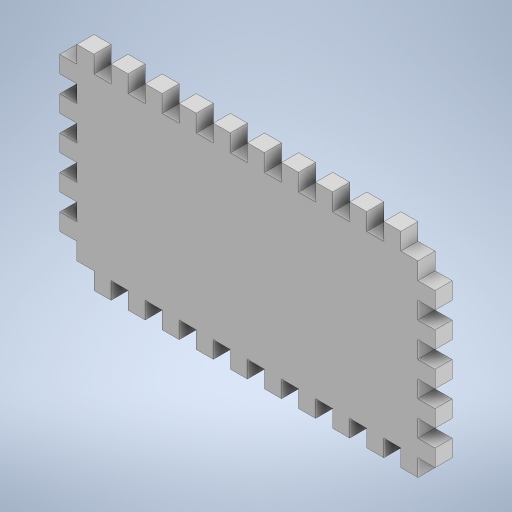
# Autodesk Inventor part: backside
Saved by Autodesk Inventor 2024 (Build 280153000, 153)
## iProperties
Created: 2024-04-15
Part Number: backside
Material: Generic
Document SubType Name: Modeling
Designer: srika
Density: 1 g/cm^3
Appearance: Default
Author: srika
Autodesk Inventor part; units mm, degrees
ref_plane "YZ Plane" through (0, 0, 0) normal (1, 0, 0) x (0, 1, 0)
ref_plane "XZ Plane" through (0, 0, 0) normal (0, 1, 0) x (-1, 0, 0)
ref_plane "XY Plane" through (0, 0, 0) normal (0, 0, 1) x (1, 0, 0)
sketch "Sketch2" plane through (0, 0, 0) normal (0, 0, 1) x (1, 0, 0)
  line L0 (0, 0) -> (5, 0)
  line L1 (5, 0) -> (5, 5)
  line L2 (5, 5) -> (0, 5)
  line L3 (0, 5) -> (0, 0)
  line L4 (5, 5) -> (105, 5)
  line L5 (105, 5) -> (105, 55)
  line L6 (105, 55) -> (5, 55)
  line L7 (5, 55) -> (5, 5)
  line L8 (105, 55) -> (110, 55)
  line L9 (110, 55) -> (110, 60)
  line L10 (110, 60) -> (105, 60)
  line L11 (105, 60) -> (105, 55)
  line L12 (100, 60) -> (95, 60)
  line L13 (100, 55) -> (100, 60)
  line L14 (95, 60) -> (95, 55)
  line L15 (90, 60) -> (85, 60)
  line L16 (90, 55) -> (90, 60)
  line L17 (85, 60) -> (85, 55)
  line L18 (80, 60) -> (75, 60)
  line L19 (80, 55) -> (80, 60)
  line L20 (75, 60) -> (75, 55)
  line L21 (70, 60) -> (65, 60)
  line L22 (70, 55) -> (70, 60)
  line L23 (65, 60) -> (65, 55)
  line L24 (60, 60) -> (55, 60)
  line L25 (60, 55) -> (60, 60)
  line L26 (55, 60) -> (55, 55)
  line L27 (50, 60) -> (45, 60)
  line L28 (50, 55) -> (50, 60)
  line L29 (45, 60) -> (45, 55)
  line L30 (40, 60) -> (35, 60)
  line L31 (40, 55) -> (40, 60)
  line L32 (35, 60) -> (35, 55)
  line L33 (30, 60) -> (25, 60)
  line L34 (30, 55) -> (30, 60)
  line L35 (25, 60) -> (25, 55)
  line L36 (20, 60) -> (15, 60)
  line L37 (20, 55) -> (20, 60)
  line L38 (15, 60) -> (15, 55)
  line L39 (10, 60) -> (5, 60)
  line L40 (10, 55) -> (10, 60)
  line L41 (5, 60) -> (5, 55)
  line L42 (105, 50) -> (105, 45)
  line L43 (110, 45) -> (110, 50)
  line L44 (110, 50) -> (105, 50)
  line L45 (105, 45) -> (110, 45)
  line L46 (105, 40) -> (105, 35)
  line L47 (110, 35) -> (110, 40)
  line L48 (110, 40) -> (105, 40)
  line L49 (105, 35) -> (110, 35)
  line L50 (105, 30) -> (105, 25)
  line L51 (110, 25) -> (110, 30)
  line L52 (110, 30) -> (105, 30)
  line L53 (105, 25) -> (110, 25)
  line L54 (105, 20) -> (105, 15)
  line L55 (110, 15) -> (110, 20)
  line L56 (110, 20) -> (105, 20)
  line L57 (105, 15) -> (110, 15)
  line L58 (105, 10) -> (105, 5)
  line L59 (110, 5) -> (110, 10)
  line L60 (110, 10) -> (105, 10)
  line L61 (105, 5) -> (110, 5)
  line L62 (0, 10) -> (5, 10)
  line L63 (5, 10) -> (5, 15)
  line L64 (5, 15) -> (0, 15)
  line L65 (0, 15) -> (0, 10)
  line L66 (0, 20) -> (5, 20)
  line L67 (5, 20) -> (5, 25)
  line L68 (5, 25) -> (0, 25)
  line L69 (0, 25) -> (0, 20)
  line L70 (0, 30) -> (5, 30)
  line L71 (5, 30) -> (5, 35)
  line L72 (5, 35) -> (0, 35)
  line L73 (0, 35) -> (0, 30)
  line L74 (0, 40) -> (5, 40)
  line L75 (5, 40) -> (5, 45)
  line L76 (5, 45) -> (0, 45)
  line L77 (0, 45) -> (0, 40)
  line L78 (0, 50) -> (5, 50)
  line L79 (5, 50) -> (5, 55)
  line L80 (5, 55) -> (0, 55)
  line L81 (0, 55) -> (0, 50)
  line L82 (15, 5) -> (10, 5)
  line L83 (10, 0) -> (15, 0)
  line L84 (15, 0) -> (15, 5)
  line L85 (10, 5) -> (10, 0)
  line L86 (25, 5) -> (20, 5)
  line L87 (20, 0) -> (25, 0)
  line L88 (25, 0) -> (25, 5)
  line L89 (20, 5) -> (20, 0)
  line L90 (35, 5) -> (30, 5)
  line L91 (30, 0) -> (35, 0)
  line L92 (35, 0) -> (35, 5)
  line L93 (30, 5) -> (30, 0)
  line L94 (45, 5) -> (40, 5)
  line L95 (40, 0) -> (45, 0)
  line L96 (45, 0) -> (45, 5)
  line L97 (40, 5) -> (40, 0)
  line L98 (55, 5) -> (50, 5)
  line L99 (50, 0) -> (55, 0)
  line L100 (55, 0) -> (55, 5)
  line L101 (50, 5) -> (50, 0)
  line L102 (65, 5) -> (60, 5)
  line L103 (60, 0) -> (65, 0)
  line L104 (65, 0) -> (65, 5)
  line L105 (60, 5) -> (60, 0)
  line L106 (75, 5) -> (70, 5)
  line L107 (70, 0) -> (75, 0)
  line L108 (75, 0) -> (75, 5)
  line L109 (70, 5) -> (70, 0)
  line L110 (85, 5) -> (80, 5)
  line L111 (80, 0) -> (85, 0)
  line L112 (85, 0) -> (85, 5)
  line L113 (80, 5) -> (80, 0)
  line L114 (95, 5) -> (90, 5)
  line L115 (90, 0) -> (95, 0)
  line L116 (95, 0) -> (95, 5)
  line L117 (90, 5) -> (90, 0)
  line L118 (105, 5) -> (100, 5)
  line L119 (100, 0) -> (105, 0)
  line L120 (105, 0) -> (105, 5)
  line L121 (100, 5) -> (100, 0)
  circle A0 centre (12.3298, 40) radius 3.5
  line L122 (6.3298, 15) -> (18.3298, 15)
  line L123 (18.3298, 15) -> (18.3298, 45)
  line L124 (18.3298, 45) -> (6.3298, 45)
  line L125 (6.3298, 45) -> (6.3298, 15)
  line L126 (6.3298, 15) -> (18.3298, 45) construction
  line L127 (18.3298, 15) -> (6.3298, 45) construction
  line L128 (19, 15) -> (31, 15)
  circle A1 centre (25, 40) radius 3.5
  line L129 (19, 45) -> (19, 15)
  line L130 (31, 15) -> (31, 45)
  line L131 (19, 15) -> (31, 45) construction
  line L132 (31, 15) -> (19, 45) construction
  line L133 (31, 45) -> (19, 45)
  line L134 (31.5, 15) -> (43.5, 15)
  circle A2 centre (37.5, 40) radius 3.5
  line L135 (31.5, 45) -> (31.5, 15)
  line L136 (43.5, 15) -> (43.5, 45)
  line L137 (31.5, 15) -> (43.5, 45) construction
  line L138 (43.5, 15) -> (31.5, 45) construction
  line L139 (43.5, 45) -> (31.5, 45)
  line L140 (44.1702, 45) -> (44.1702, 15)
  line L141 (56.1702, 15) -> (56.1702, 45)
  line L142 (56.1702, 15) -> (44.1702, 45) construction
  line L143 (44.1702, 15) -> (56.1702, 45) construction
  line L144 (56.1702, 45) -> (44.1702, 45)
  circle A3 centre (50.1702, 40) radius 3.5
  line L145 (44.1702, 15) -> (56.1702, 15)
  line L146 (57.3642, 14.8119) -> (69.3642, 14.8119)
  line L147 (57.3642, 44.8119) -> (57.3642, 14.8119)
  line L148 (69.3642, 44.8119) -> (57.3642, 44.8119)
  line L149 (57.3642, 14.8119) -> (69.3642, 44.8119) construction
  line L150 (69.3642, 14.8119) -> (57.3642, 44.8119) construction
  line L151 (69.3642, 14.8119) -> (69.3642, 44.8119)
  circle A4 centre (63.3642, 39.8119) radius 3.5
  line L152 (75, 15) -> (100, 15)
  line L153 (100, 15) -> (100, 45)
  line L154 (100, 45) -> (75, 45)
  line L155 (75, 45) -> (75, 15)
  line L156 (75, 15) -> (100, 45) construction
  line L157 (100, 15) -> (75, 45) construction
  line L158 (82.75, 38.25) -> (92.25, 38.25)
  line L159 (92.25, 38.25) -> (92.25, 41.75)
  line L160 (92.25, 41.75) -> (82.75, 41.75)
  line L161 (82.75, 41.75) -> (82.75, 38.25)
  line L162 (82.75, 38.25) -> (92.25, 41.75) construction
  line L163 (92.25, 38.25) -> (82.75, 41.75) construction
  point P0 (87.5, 30)
  point P1 (87.5, 40)
  dimension "d0" = 5
  dimension "d1" = 5
  dimension "d4" = 5
  dimension "d5" = 5
  dimension "d8" = 10
  dimension "d15" = 10
  dimension "d22" = 10
  dimension "d29" = 10
  dimension "d37" = 7
  dimension "d38" = 12
  dimension "d39" = 30
  dimension "d51" = 7
  dimension "d52" = 12
  dimension "d53" = 30
  dimension "d54" = 7
  dimension "d55" = 12
  dimension "d56" = 30
  dimension "d57" = 7
  dimension "d58" = 12
  dimension "d59" = 30
  dimension "d60" = 7
  dimension "d61" = 12
  dimension "d62" = 30
  dimension "d63" = 25
  dimension "d64" = 30
  dimension "d65" = 9.5
  dimension "d66" = 3.5
  constraints: 324 end point, 80 horizontal alignment, 59 parallel, 30 collinear, 9 horizontal, 9 perpendicular, 5 centre point, 4 midpoint, 3 vertical, 86 other
  measures "d0" distance of L2.end L1.end
  measures "d1" distance of L1.end L0.end
  measures "d4" distance of L10.end L9.end
  measures "d5" distance of L9.end L8.end
  measures "d8" distance of L9.end L12.start
  measures "d15" distance of L5.end L42.end
  measures "d22" distance of L1.end L63.end
  measures "d29" distance of L2.end L82.end
  measures "d37" diameter of A0
  measures "d38" distance of L125.start L123.end
  measures "d39" distance of L123.end L122.end
  measures "d51" diameter of A1
  measures "d52" distance of L129.start L130.end
  measures "d53" distance of L130.end L130.start
  measures "d54" diameter of A2
  measures "d55" distance of L139.end L136.end
  measures "d56" distance of L136.end L136.start
  measures "d57" diameter of A3
  measures "d58" distance of L140.start L144.start
  measures "d59" distance of L144.start L145.end
  measures "d60" diameter of A4
  measures "d61" distance of L147.start L148.start
  measures "d62" distance of L148.start L146.end
  measures "d63" distance of L154.end L153.end
  measures "d64" distance of L153.end L152.end
  measures "d65" distance of L160.end L159.end
  measures "d66" distance of L159.end L158.end
extrude "Extrusion1" add sketch "Sketch2" along normal blind 5 contours L7 L6 L5 L4 | L4 L84 L83 L85 | L62 L65 L64 L7 | L4 L88 L87 L89 | L66 L69 L68 L7 | L4 L92 L91 L93 | L70 L73 L72 L7 | L4 L96 L95 L97 | L74 L77 L76 L7 | L4 L100 L99 L101 | L78 L81 L80 L7 | L41 L39 L40 L6 | L4 L104 L103 L105 | L38 L36 L37 L6 | L4 L108 L107 L109 | L35 L33 L34 L6 | L4 L112 L111 L113 | L32 L30 L31 L6 | L4 L116 L115 L117 | L29 L27 L28 L6 | L4 L120 L119 L121 | L5 L60 L59 L61 | L26 L24 L25 L6 | L5 L56 L55 L57 | L23 L21 L22 L6 | L5 L52 L51 L53 | L20 L18 L19 L6 | L5 L48 L47 L49 | L17 L15 L16 L6 | L5 L44 L43 L45 | L14 L12 L13 L6 | A0 | L125 L124 L123 L122 | L129 L133 L130 L128 | A1 | L135 L139 L136 L134 | A2 | L144 L141 L145 L140 | A3 | L147 L148 L151 L146 | A4 | L155 L154 L153 L152 | L161 L160 L159 L158
body "Solid1"
